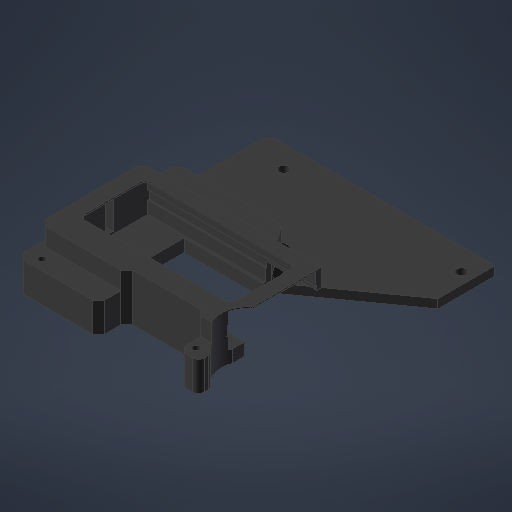
# Autodesk Inventor part: screen_top
Saved by Autodesk Inventor 2026.1 (Build 301233000, 233)
## iProperties
Created: 2026-07-03
Part Number: screen_top
Material: Generic
Document SubType Name: Modeling
Designer: aaron
Density: 1 g/cm^3
Appearance: Default
Author: aaron
Autodesk Inventor part; units mm, degrees
ref_plane "YZ Plane" through (0, 0, 0) normal (1, 0, 0) x (0, 1, 0)
ref_plane "XZ Plane" through (0, 0, 0) normal (0, 1, 0) x (-1, 0, 0)
ref_plane "XY Plane" through (0, 0, 0) normal (0, 0, 1) x (1, 0, 0)
sketch "Sketch1" plane through (0, 0, 0) normal (0, 1, 0) x (-1, 0, 0)
  line L0 (0, 0) -> (84, 0)
  line L1 (84, 0) -> (84, -50)
  line L2 (84, -50) -> (0, -50)
  line L3 (0, -50) -> (0, 0)
  line L4 (80, -15) -> (27, -15)
  line L5 (27, -15) -> (27, -39.3)
  line L6 (27, -39.3) -> (80, -39.3)
  line L7 (80, -39.3) -> (80, -15)
  dimension "d0" = 50
  dimension "d1" = 84
  dimension "d2" = 53
  dimension "d3" = 24.3
  dimension "d4" = 4
  dimension "d5" = 15
  constraints: 16 end point, 4 parallel, 2 horizontal, 2 perpendicular
  measures "d0" distance of L0.end L1.end
  measures "d1" distance of L0.start L0.end
  measures "d2" distance of L4.start L4.end
  measures "d3" distance of L4.end L5.end
  measures "d4" distance between parallel lines of L1 L7
  measures "d5" distance between parallel lines of L0 L4
extrude "Extrusion1" add sketch "Sketch1" along normal blind 16
sketch "Sketch2" plane through (0, 16, 0) normal (0, 1, 0) x (1, 0, 0)
  ellipse E0 centre (-18.075, 11.895) end of major axis (-18.075, 2.995) minor radius 8.9 projected
  line L0 (-22.7777, 4.3389) -> (-22.7777, -5.9825)
  line L1 (-84, 0) -> (0, 0) projected
  line L2 (-22.7777, -5.9825) -> (6.1455, -5.9825)
  line L3 (6.1455, -5.9825) -> (6.1455, 53.3194)
  line L4 (6.1455, 53.3194) -> (-6.2419, 53.3194)
  line L5 (-6.2419, 53.3194) -> (-6.2419, 41.6355)
  line L6 (-23.8443, 18.6718) -> (-6.2419, 41.6355)
  constraints: 12 end point, 5 perpendicular, 3 other
sketch "Sketch3" plane through (0, 16, 0) normal (0, 1, 0) x (1, 0, 0)
  ellipse E0 centre (-78.9717, 3.5) end of major axis (-78.9717, 1.85) minor radius 1.65 projected
  ellipse E1 centre (-26.9717, 3.5) end of major axis (-26.9717, 1.85) minor radius 1.65 projected
  ellipse E2 centre (-11.4931, 46.5) end of major axis (-11.4931, 44.35) minor radius 2.15 projected
  ellipse E3 centre (-71.4931, 46.5) end of major axis (-71.4931, 44.35) minor radius 2.15 projected
  circle A0 centre (-78.9717, 3.5) radius 1.15
  circle A1 centre (-71.4931, 46.5) radius 1.65
  circle A2 centre (-11.4931, 46.5) radius 1.65
  circle A3 centre (-26.9717, 3.5) radius 1.15
  point P0 (0, 0)
  dimension "d25" = 2.3
  dimension "d26" = 3.3
  dimension "d27" = 3.3
  dimension "d28" = 2.3
  constraints: 4 centre point, 4 coincident
  measures "d25" diameter of A0
  measures "d26" diameter of A1
  measures "d27" diameter of A2
  measures "d28" diameter of A3
sketch "Sketch4" plane through (0, 0, 0) normal (1, 0, 0) x (0, 0, -1)
  line L0 (15, 0) -> (15, 16) projected
  line L1 (39.3, 0) -> (39.3, 16) projected
  line L2 (14.15, 15.5) -> (40.15, 15.5)
  line L3 (40.15, 15.5) -> (40.15, 4.25)
  line L4 (40.15, 4.25) -> (14.15, 4.25)
  line L5 (14.15, 4.25) -> (14.15, 15.5)
  line L6 (0, 16) -> (50, 16) projected
  line L7 (13.65, 11.4) -> (40.65, 11.4)
  line L8 (40.65, 11.4) -> (40.65, 8.4)
  line L9 (40.65, 8.4) -> (13.65, 8.4)
  line L10 (13.65, 8.4) -> (13.65, 11.4)
  point P0 (0, 0)
  point P1 (39.3, 11.4)
  point P2 (39.3, 15.5)
  point P3 (14.15, 11.4)
  point P4 (14.15, 8.4)
  point P5 (40.15, 8.4)
  point P6 (40.15, 11.4)
  dimension "d8" = 0.5
  dimension "d9" = 27
  dimension "d10" = 26
  dimension "d11" = 0.5
  dimension "d12" = 11.25
  dimension "d13" = 0.85
  dimension "d16" = 4.1
  dimension "d17" = 3
  constraints: 16 end point, 4 parallel, 2 horizontal, 2 perpendicular
  measures "d8" distance between parallel lines of L6 L2
  measures "d9" distance of L8.end L9.end
  measures "d10" distance of L3.end L4.end
  measures "d11" distance between parallel lines of L5 L10
  measures "d12" distance of L2.end L3.end
  measures "d13" distance between parallel lines of L5 L0
  measures "d16" distance between parallel lines of L2 L7
  measures "d17" distance between parallel lines of L7 L9
extrude "Extrusion2" cut sketch "Sketch4" against normal up to surface (80 mm away) contours L4 L5 L9 L0 | L0 L9 L1 L4 | L9 L5 L7 L0 | L0 L7 L1 L9 | L1 L9 L3 L4 | L7 L5 L2 L0 | L0 L2 L1 L7 | L1 L7 L3 L9 | L9 L10 L7 L5 | L1 L2 L3 L7 | L3 L7 L8 L9
sketch "Sketch5" plane through (0, 16, 0) normal (0, 1, 0) x (1, 0, 0)
  line L0 (-27, 15) -> (-80, 15) projected
  line L1 (-80, 15) -> (-80, 39.3) projected
  line L2 (-80, 39.3) -> (-27, 39.3) projected
  line L3 (-27, 39.3) -> (-27, 15) projected
  line L4 (-77, 16) -> (-30, 16)
  line L5 (-28, 18) -> (-28, 36.3)
  line L6 (-30, 38.3) -> (-77, 38.3)
  line L7 (-79, 36.3) -> (-79, 18)
  arc A0 (-79, 18) -> (-77, 16) centre (-77, 18) ccw
  arc A1 (-77, 38.3) -> (-79, 36.3) centre (-77, 36.3) ccw
  arc A2 (-28, 36.3) -> (-30, 38.3) centre (-30, 36.3) ccw
  arc A3 (-30, 16) -> (-28, 18) centre (-30, 18) ccw
  point P0 (0, 0)
  dimension "d18" = 1
  dimension "d19" = 2
  constraints: 8 end point, 8 point on circle, 8 tangent, 4 centre point, 3 equal radius, 3 other
  measures "d18" distance between parallel lines of L0 L4
  measures "d19" radius of A0
extrude "Extrusion3" add sketch "Sketch5" against normal blind 0.5
extrude "Extrusion4" cut sketch "Sketch2" against normal through all
fillet "Fillet1" radius 2 4 edges at (-6.2419, 8, -50) (-22.7777, 8, 0) (-22.7777, 8, -4.3389) (-6.2419, 8, -41.6355)
extrude "Extrusion5" cut sketch "Sketch3" against normal through all contours A0 | A1 | A2 | A3
sketch "Sketch6" plane through (0, 16, 0) normal (0, 1, 0) x (1, 0, 0)
  line L0 (-86.9159, -3.2646) -> (-13.006, -3.2646)
  line L1 (-13.006, -3.2646) -> (-13.006, 7.5477)
  line L2 (-13.006, 7.5477) -> (-86.9159, 7.5477)
  line L3 (-86.9159, 7.5477) -> (-86.9159, -3.2646)
  line L4 (-87.4382, 54.3485) -> (-2.9773, 54.3485)
  line L5 (-2.9773, 54.3485) -> (-2.9773, 42.2985)
  line L6 (-2.9773, 42.2985) -> (-87.4382, 42.2985)
  line L7 (-87.4382, 42.2985) -> (-87.4382, 54.3485)
  point P0 (0, 0)
  constraints: 16 end point, 4 parallel, 2 horizontal, 2 perpendicular
extrude "Extrusion6" cut sketch "Sketch6" against normal blind 6
chamfer "Chamfer1" distance 2 angle 45 3 edges at (-84, 5, 0) (-84, 13, -42.2985) (-84, 13, -7.5477)
sketch "Sketch7" plane through (0, 0, 0) normal (0, -1, 0) x (1, 0, 0)
  line L0 (-27, -15) -> (-80, -15) projected
  line L1 (-80, -15) -> (-80, -39.3) projected
  line L2 (-80, -39.3) -> (-27, -39.3) projected
  line L3 (-66.9548, -15) -> (-66.9548, -39.3)
  point P0 (0, 0)
  constraints: 2 end point, 2 point on line, 1 perpendicular
extrude "Extrusion7" add sketch "Sketch7" against normal up to surface (4.25 mm away)
sketch "Sketch8" plane through (-80, 4.25, -14.15) normal (0, 1, 0) x (1, 0, 0)
  line L0 (53, 0.85) -> (13.0452, 0.85) projected
  line L1 (50.7563, 0.85) -> (67.3489, 0.85)
  line L2 (67.3489, 0.85) -> (67.3489, 12.5038)
  line L3 (67.3489, 12.5038) -> (50.7563, 12.5038)
  line L4 (50.7563, 12.5038) -> (50.7563, 0.85)
  point P0 (80, -14.15)
  point P1 (53, 0.85)
  constraints: 8 end point, 2 parallel, 1 horizontal, 1 perpendicular, 1 point on line
extrude "Extrusion8" cut sketch "Sketch8" against normal through all
sketch "Sketch9" plane through (0, 16, 0) normal (0, 1, 0) x (1, 0, 0)
  line L0 (-23.5001, 14.9994) -> (-4.4637, 14.9994)
  line L1 (-4.4637, 14.9994) -> (-4.4637, 54.7132)
  line L2 (-4.4637, 54.7132) -> (-23.5001, 54.7132)
  line L3 (-23.5001, 54.7132) -> (-23.5001, 14.9994)
  point P0 (0, 0)
  constraints: 8 end point, 2 parallel, 1 horizontal, 1 perpendicular
extrude "Extrusion9" cut sketch "Sketch9" against normal through all
sketch "Sketch10" plane through (-80, 4.25, -14.15) normal (0, 1, 0) x (1, 0, 0)
  line L0 (13.0452, 25.15) -> (53, 25.15) projected
  line L1 (51.4728, 25.15) -> (61.1436, 25.15)
  line L2 (61.1436, 25.15) -> (61.1436, 10.3359)
  line L3 (61.1436, 10.3359) -> (51.4728, 10.3359)
  line L4 (51.4728, 10.3359) -> (51.4728, 25.15)
  point P0 (80, -14.15)
  point P1 (53, 25.15)
  constraints: 8 end point, 2 parallel, 1 horizontal, 1 perpendicular, 1 point on line
extrude "Extrusion10" cut sketch "Sketch10" against normal through all
sketch "Sketch11" plane through (0, 0, 0) normal (0, -1, 0) x (1, 0, 0)
  line L0 (-26.4158, -15) -> (-66.9548, -15) projected
  line L1 (-26.4158, -15) -> (-34.9227, -15)
  line L2 (-34.9227, -15) -> (-34.9227, -19)
  line L3 (-34.9227, -19) -> (-26.4158, -19)
  line L4 (-26.4158, -19) -> (-26.4158, -15)
  point P0 (0, 0)
  dimension "d49" = 4
  constraints: 8 end point, 2 parallel, 1 horizontal, 1 perpendicular
  measures "d49" distance between parallel lines of L0 L3
extrude "Extrusion11" add sketch "Sketch11" against normal up to surface (4.25 mm away)
chamfer "Chamfer3" distance 4 angle 45 1 edges at (-34.9227, 2.125, -15)
sketch "Sketch12" plane through (0, 0, 0) normal (0, -1, 0) x (1, 0, 0)
  line L0 (-20.2339, -35.0747) -> (-40.3579, -35.0747)
  line L1 (-40.3579, -35.0747) -> (-40.3579, -55.8547)
  line L2 (-40.3579, -55.8547) -> (-20.2339, -55.8547)
  line L3 (-20.2339, -55.8547) -> (-20.2339, -35.0747)
  point P0 (0, 0)
  constraints: 8 end point, 2 parallel, 1 horizontal, 1 perpendicular
extrude "Extrusion12" cut sketch "Sketch12" against normal up to surface (10 mm away)
sketch "Sketch13" plane through (-84, 0, -50) normal (0, 0, -1) x (-1, 0, 0)
  line L0 (-43.6421, 10) -> (-43.6421, 0) projected
  line L1 (-43.6421, 0) -> (0, 0) projected
  line L2 (0, 0) -> (0, 10) projected
  line L3 (0, 10) -> (-43.6421, 10) projected
  point P0 (-84, 0)
extrude "Extrusion13" add sketch "Sketch13" along normal blind 34.9
sketch "Sketch14" plane through (0, 10, 0) normal (0, 1, 0) x (1, 0, 0)
  ellipse E0 centre (-71.4931, 77.55) end of major axis (-71.4931, 75.4) minor radius 2.15 projected
  circle A0 centre (-71.4931, 77.55) radius 1.65
  point P0 (0, 0)
  dimension "d57" = 3.3
  constraints: 1 centre point, 1 coincident
  measures "d57" diameter of A0
extrude "Extrusion14" cut sketch "Sketch14" against normal through all contours A0
chamfer "Chamfer5" distance 2 angle 45 1 edges at (-84, 5, -84.9)
sketch "Sketch15" plane through (-80, 4.25, -40.15) normal (1, 0, 0) x (0, 0, -1)
  line L0 (-14.1662, 10.293) -> (-11.6439, 10.293)
  line L1 (-11.6439, 10.293) -> (-11.6439, 0.8492)
  line L2 (-11.6439, 0.8492) -> (-14.1662, 0.8492)
  line L3 (-14.1662, 0.8492) -> (-14.1662, 10.293)
  point P0 (-40.15, -4.25)
  constraints: 8 end point, 2 parallel, 1 horizontal, 1 perpendicular
extrude "Extrusion15" cut sketch "Sketch15" against normal through all
sketch "Sketch16" plane through (0, 16, 0) normal (0, 1, 0) x (1, 0, 0)
  line L0 (-48.0667, 2.12) -> (-48.0667, 6.12) projected
  line L1 (-37.9167, 2.12) -> (-48.0667, 2.12) projected
  line L2 (-37.9167, 6.12) -> (-37.9167, 2.12) projected
  line L3 (-56.4917, -25.4613) -> (-29.4917, -25.4613)
  line L4 (-29.4917, -25.4613) -> (-29.4917, 7.5477)
  line L5 (-31.4917, 9.5477) -> (-54.4917, 9.5477)
  line L6 (-56.4917, 7.5477) -> (-56.4917, -25.4613)
  line L7 (-82, 7.5477) -> (-25.841, 7.5477) projected
  line L8 (-37.9167, 2.12) -> (-29.4917, 2.12)
  line L9 (-48.0667, 2.12) -> (-56.4917, 2.12)
  line L10 (-56.4917, 7.5477) -> (-54.4917, 9.5477)
  line L11 (-29.4917, 7.5477) -> (-31.4917, 9.5477)
  point P0 (0, 0)
  point P1 (-29.4917, 9.5477)
  point P2 (-56.4917, 9.5477)
  dimension "d69" = 27
  dimension "d71" = 2
  dimension "d72" = 2
  dimension "d73" = 2
  dimension "d74" = 2
  dimension "d75" = 2
  constraints: 16 end point, 7 point on line, 2 parallel, 2 perpendicular, 1 collinear, 1 horizontal
  measures "d69" distance of L3.start L3.end
  measures "d71" distance between parallel lines of L5 L7
  measures "d72" distance of L6.start point (-56.492, 9.548)
  measures "d73" distance of L5.end point (-56.492, 9.548)
  measures "d74" distance of L4.end point (-29.492, 9.548)
  measures "d75" distance of L5.start point (-29.492, 9.548)
extrude "Extrusion16" cut sketch "Sketch16" against normal through all
chamfer "Chamfer6" distance 2 angle 45 2 edges at (-56.4917, 5, 0) (-29.4917, 5, 0)
sketch "Sketch17" plane through (0, 10, 0) normal (0, 1, 0) x (1, 0, 0)
  line L0 (-40.3579, 84.9) -> (-7.6346, 84.9)
  line L1 (-7.6346, 84.9) -> (-7.6346, 65.6879)
  line L2 (-7.6346, 65.6879) -> (-40.3579, 65.6879)
  line L3 (-40.3579, 65.6879) -> (-40.3579, 84.9)
  line L4 (-23.5001, 42.2985) -> (-82, 42.2985) projected
  line L5 (-40.3579, 42.2985) -> (-7.6346, 65.6879)
  line L6 (-40.3579, 84.9) -> (-40.3579, 39.3) projected
  line L7 (-40.3579, 84.9) -> (-40.3579, 42.2985)
  ellipse E0 centre (-11.4931, 77.55) end of major axis (-11.4931, 75.4) minor radius 2.15 projected
  circle A0 centre (-11.4931, 77.55) radius 1.65
  point P0 (0, 0)
  dimension "d81" = 3.3
  constraints: 12 end point, 2 parallel, 1 centre point, 1 coincident, 1 collinear, 1 horizontal, 1 perpendicular, 1 point on line
  measures "d81" diameter of A0
extrude "Extrusion17" add sketch "Sketch17" against normal blind 10 contours L0 L1 L2 L3 | L2 L5 L6 | E0
sketch "Sketch18" plane through (0, 10, 0) normal (0, 1, 0) x (1, 0, 0)
  circle A0 centre (-11.4931, 77.55) radius 1.65 projected
  line L0 (-84, 82.9) -> (-82, 84.9) projected
  line L1 (-84, 40.2985) -> (-84, 82.9) projected
  line L2 (-82, 42.2985) -> (-84, 40.2985) projected
  line L3 (-40.3579, 42.2985) -> (-82, 42.2985) projected
  line L4 (-40.3579, 42.2985) -> (-7.6346, 65.6879) projected
  line L5 (-7.6346, 65.6879) -> (-7.6346, 84.9) projected
  line L6 (-82, 84.9) -> (-7.6346, 84.9) projected
  circle A1 centre (-71.4931, 77.55) radius 1.65 projected
  circle A2 centre (-71.4931, 46.5) radius 1.65 projected
  line L7 (-40.3579, 42.2985) -> (-48.7168, 53.9932)
  line L8 (-48.7168, 53.9932) -> (-84, 53.9932)
  point P0 (0, 0)
  constraints: 4 end point, 1 perpendicular, 1 point on line
extrude "Extrusion18" cut sketch "Sketch18" against normal blind 7 contours L0 L6 L5 L4 L7 L8 L1
chamfer "Chamfer7" distance 2 angle 45 3 edges at (-44.5374, 3, -48.1458) (-66.3584, 3, -53.9932) (-84, 6.5, -53.9932)
equation "\"d73\" = d72"
equation "\"d74\" = d72"
equation "\"d75\" = d74"
body "Solid1"
